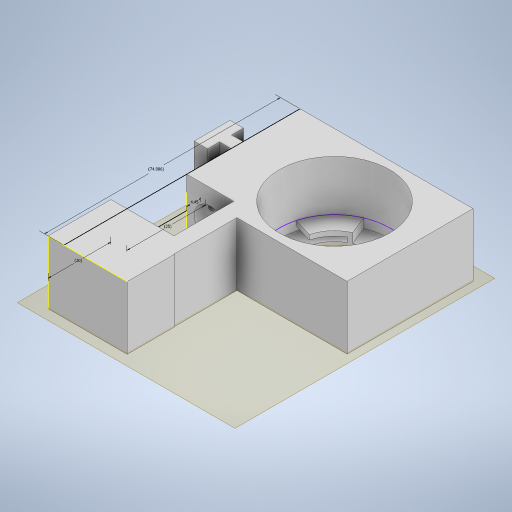
# Autodesk Inventor part: spoutextrusion
Saved by Autodesk Inventor 2023 (Build 270158000, 158)
## iProperties
Created: 2025-10-02
Part Number: spoutextrusion
Material: Generic
Document SubType Name: Modeling
Designer: ptato_qo49uko
Density: 1 g/cm^3
Appearance: Default
Author: ptato_qo49uko
Autodesk Inventor part; units mm, degrees
ref_plane "YZ Plane" through (0, 0, 0) normal (1, 0, 0) x (0, 1, 0)
ref_plane "XZ Plane" through (0, 0, 0) normal (0, 1, 0) x (-1, 0, 0)
ref_plane "XY Plane" through (0, 0, 0) normal (0, 0, 1) x (1, 0, 0)
sketch "Sketch1" plane through (0, 0, 0) normal (0, 1, 0) x (-1, 0, 0)
  line L0 (-2.2478, 1.8858) -> (1.3522, 1.8858)
  line L1 (-2.2478, 1.8858) -> (-2.2478, -1.9142)
  line L2 (-2.2478, -1.9142) -> (1.3522, -1.9142)
  line L3 (1.3522, 1.8858) -> (1.3522, 5.6858)
  line L4 (1.3522, -1.9142) -> (1.3522, -5.7142)
  line L5 (1.3522, -5.7142) -> (5.6322, -5.7142)
  line L6 (5.6322, -5.7142) -> (5.6322, 5.6858)
  line L7 (1.3522, 5.6858) -> (5.6322, 5.6858)
  point P0 (0, 0)
  dimension "d1" = 3.6
  dimension "d2" = 3.8
  dimension "d3" = 3.8
  dimension "d4" = 3.8
  dimension "d6" = 4.28
  dimension "d7" = 11.4
  dimension "d98" = 3.6
  constraints: 16 end point, 3 vertical, 2 horizontal, 2 perpendicular
  measures "d1" distance of L0.start L0.end
  measures "d2" distance of L0.start L1.end
  measures "d3" distance of L0.end L3.end
  measures "d4" distance of L2.end L4.end
  measures "d6" distance of L4.end L5.end
  measures "d7" distance of L5.end L6.end
  measures "d98" distance of L1.end L2.end
extrude "Extrusion1" add sketch "Sketch1" along normal blind 20
sketch "Sketch2" plane through (2.2478, 0, 1.8858) normal (1, 0, 0) x (0, 0, -1)
  line L0 (3.8, 0) -> (7.6, 0) projected
  line L1 (0, 20) -> (3.8, 20) projected
  line L2 (1.9, 20) -> (-18.1, 20)
  line L3 (21.9, 20) -> (1.9, 20)
  line L4 (1.8858, 0) -> (21.8858, 0)
  line L5 (0, 0) -> (3.8, 0) projected
  line L6 (1.8858, 0) -> (-18.1, 0)
  line L7 (-18.1, 0) -> (-18.1, 20)
  line L8 (21.9, 20) -> (21.8858, 0)
  point P0 (12, 0)
  point P1 (3.8, 0)
  dimension "d17" = 20
  dimension "d26" = 20
  dimension "d27" = 20
  constraints: 12 end point, 3 point on line, 2 collinear, 1 midpoint, 1 perpendicular
  measures "d17" distance of L2.start L2.end
  measures "d26" distance of L3.start L2.start
  measures "d27" distance of L4.start L4.end
extrude "Extrusion2" add sketch "Sketch2" along normal blind 55
sketch "Sketch4" plane through (0, 20, 0) normal (0, 1, 0) x (1, 0, 0)
  line L0 (2.2478, 1.9142) -> (-1.3522, 1.9142) projected
  line L1 (2.2478, -1.8858) -> (2.2478, 1.9142)
  line L2 (2.2478, 0.0142) -> (33.2478, 0.0142)
  point P0 (0, 0)
  dimension "d16" = 31
  constraints: 4 end point, 1 horizontal, 1 midpoint, 1 vertical
  measures "d16" distance of L2.start L2.end
sketch "Sketch5" plane through (0, 20, 0) normal (0, 1, 0) x (1, 0, 0)
  point P0 (0, 0)
hole "Hole2" at (33.2478, 20, -0.0142) direction (0, -1, 0) diameter 22.5 depth 22.5 counterbore diameter 35 counterbore depth 19
sketch "Sketch6" plane through (0, 0, 0) normal (0, -1, 0) x (1, 0, 0)
  point P0 (0, 0)
sketch "Sketch7" plane through (2.2478, 0, 19.9858) normal (0, 0, 1) x (1, 0, 0)
  line L0 (0, 0) -> (55, 0) projected
  line L1 (0, 0) -> (55, 0) projected
  line L2 (15, 0) -> (15, 20)
  line L3 (15, 20) -> (20, 20)
  line L4 (0, 20) -> (55, 20) projected
  line L5 (20, 20) -> (20, 0)
  line L6 (42.25, 0) -> (19.75, 0) projected
  line L7 (15, 0) -> (20, 0)
  point P0 (-2.2478, 0)
  dimension "d41" = 5
  constraints: 8 end point, 3 point on line, 1 collinear, 1 perpendicular
  measures "d41" distance of L2.end L3.end
extrude "Extrusion4" add sketch "Sketch7" along normal blind 20
sketch "Sketch10" plane through (17.2478, 0, 19.9858) normal (-1, 0, 0) x (0, 0, 1)
  line L0 (0, 20) -> (20, 20) projected
  line L1 (0, 0) -> (20, 0) projected
  line L2 (20, 20) -> (15, 20)
  line L3 (15, 20) -> (15, 0)
  line L4 (15, 0) -> (20, 0)
  line L5 (20, 0) -> (20, 20)
  point P0 (-19.9858, 0)
  point P1 (20, 0)
  dimension "d42" = 5
  constraints: 8 end point, 2 parallel, 1 horizontal, 1 perpendicular, 1 point on line
  measures "d42" distance of L4.end L3.end
extrude "Extrusion6" add sketch "Sketch10" along normal blind 20
sketch "Sketch11" plane through (2.2478, 0, 19.9858) normal (0, 0, 1) x (1, 0, 0)
  point P0 (-2.2478, 0)
sketch "Sketch12" plane through (2.2478, 0, 19.9858) normal (0, 0, 1) x (1, 0, 0)
  point P0 (-2.2478, 0)
sketch "Sketch13" plane through (2.2478, 0, 19.9858) normal (0, 0, 1) x (1, 0, 0)
  point P0 (-2.2478, 0)
sketch "Sketch14" plane through (2.2478, 0, 19.9858) normal (0, 0, 1) x (1, 0, 0)
  line L0 (0, 0) -> (15, 0) projected
  line L1 (7.5, 0) -> (7.5, 10)
  line L2 (0, 20) -> (15, 20) projected
  point P0 (-2.2478, 0)
  dimension "d45" = 10
  constraints: 2 end point, 1 midpoint, 1 perpendicular
  measures "d45" distance of L1.start L1.end
hole "Hole3" at (9.7478, 10, 19.9858) direction (0, 0, -1) diameter 10 depth 49.5
sketch "Sketch15" plane through (2.2478, 0, 39.9858) normal (0, 0, 1) x (1, 0, 0)
  line L0 (-3.6, 20) -> (-7.88, 20) projected
  line L1 (42.25, 0) -> (19.75, 0) projected
  line L2 (-5.0624, 20) -> (20.1325, 20)
  line L3 (20.1325, 20) -> (20.1325, 0)
  line L4 (20.1325, 0) -> (-5.0624, 0)
  line L5 (20, 20) -> (-5, 20) projected
  line L6 (20, 0) -> (-5, 0) projected
  line L7 (-5, 20) -> (-5, 0)
  point P0 (-2.2478, 0)
  point P1 (19.75, 0)
  constraints: 8 end point, 2 point on line, 1 horizontal, 1 parallel, 1 perpendicular
extrude "Extrusion7" add sketch "Sketch15" along normal blind 15
sketch "Sketch18" plane through (0, 20, 0) normal (0, 1, 0) x (1, 0, 0)
  line L0 (2.2478, 1.9142) -> (2.2478, 20) projected
  line L1 (2.2478, 20) -> (2.2478, -54.9858)
  line L2 (22.3802, -54.9858) -> (-2.7522, -54.9858) projected
  point P0 (0, 0)
  dimension "d73" = 74.9858
  constraints: 2 end point, 1 point on line, 1 vertical
  measures "d73" distance of L0.end L1.end
sketch "Sketch19" plane through (2.2478, 0, 1.8858) normal (-1, 0, 0) x (0, 0, 1)
  circle A0 centre (10, 10) radius 1.55 projected
  line L0 (18.1, 20) -> (18.1, 0) projected
  line L1 (18.1, 10) -> (8.1, 10)
  point P0 (-1.8858, 0)
  dimension "d75" = 10
  constraints: 2 end point, 1 horizontal, 1 midpoint
  measures "d75" distance of L1.start L1.end
hole "Hole6" at (2.2478, 10, 9.9858) direction (1, 0, 0) diameter 3.1 depth 13.5
sketch "Sketch20" plane through (2.2478, 0, 1.8858) normal (-1, 0, 0) x (0, 0, 1)
  circle A0 centre (8.1, 10) radius 1.55 projected
  line L0 (8.1, 10) -> (33.1, 10)
  line L1 (33.1, 20) -> (33.1, 0) projected
  point P0 (-1.8858, 0)
  dimension "d83" = 25
  constraints: 2 end point, 1 midpoint
  measures "d83" distance of L0.start L0.end
sketch "Sketch21" plane through (17.2478, 0, 19.9858) normal (-1, 0, 0) x (0, 0, 1)
  point P0 (-19.9858, 0)
sketch "Sketch22" plane through (0, 20, 0) normal (0, 1, 0) x (1, 0, 0)
  line L0 (2.2478, -19.9858) -> (17.2478, -19.9858) projected
  line L1 (2.2478, -19.9858) -> (17.2478, -19.9858)
  line L2 (17.2478, -19.9858) -> (17.2478, -15.9858)
  line L3 (17.2478, -15.9858) -> (2.2478, -15.9858)
  line L4 (2.2478, -15.9858) -> (2.2478, -19.9858)
  point P0 (0, 0)
  dimension "d84" = 15
  dimension "d85" = 4
  constraints: 8 end point, 2 parallel, 1 horizontal, 1 perpendicular
  measures "d84" distance of L3.end L2.end
  measures "d85" distance of L2.end L1.end
extrude "Extrusion8" cut sketch "Sketch22" against normal blind 22.25
sketch "Sketch23" plane through (17.2478, 0, 34.9858) normal (0, 0, -1) x (-1, 0, 0)
  circle A0 centre (10, 10) radius 2.5 projected
  circle A1 centre (7.5, 10) radius 3
  point P0 (17.2478, 0)
  dimension "d88" = 6
  constraints: 1 centre point, 1 horizontal alignment, 1 other
  measures "d88" diameter of A1
hole "Hole7" at (9.7478, 10, 34.9858) direction (0, 0, 1) diameter 6 depth 17
sketch "Sketch24" plane through (2.2478, 0, 1.8858) normal (-1, 0, 0) x (0, 0, 1)
  circle A0 centre (8.1, 10) radius 1.55 projected
  line L0 (9.65, 10) -> (14.1, 10)
  line L1 (14.1, 5) -> (14.1, 15) projected
  point P0 (-1.8858, 0)
  dimension "d96" = 4.45
  constraints: 2 end point, 1 horizontal alignment, 1 midpoint, 1 other
  measures "d96" distance of L0.start L0.end
sketch "Sketch25" plane through (-2.7522, 0, 19.9858) normal (-1, 0, 0) x (0, 0, 1)
  line L0 (15, 0) -> (15, 20) projected
  line L1 (15, 10) -> (35, 10)
  line L2 (35, 0) -> (35, 20) projected
  point P0 (-19.9858, 0)
  dimension "d97" = 20
  constraints: 2 end point, 2 midpoint
  measures "d97" distance of L1.start L1.end
ref_plane "Work Plane2" through (33.2478, 0.5, -0.0142) normal (0, 1, 0) x (1, 0, 0)
sketch "Sketch26" plane through (33.2478, 1, -0.0142) normal (0, 1, 0) x (1, 0, 0)
  circle A0 centre (0, 0) radius 17.5
  point P0 (-33.2478, -0.0142)
  constraints: 1 centre point
extrude "Extrusion9" add sketch "Sketch26" along normal blind 3
sketch "Sketch27" plane through (33.2478, 4, -0.0142) normal (0, 1, 0) x (1, 0, 0)
  circle A0 centre (0, 0) radius 17.5
  point P0 (-33.2478, -0.0142)
  constraints: 1 centre point
sketch "Sketch29" plane through (33.2478, 1, -0.0142) normal (0, -1, 0) x (1, 0, 0)
  circle A0 centre (0, 0) radius 17.5
  point P0 (-33.2478, 0.0142)
  constraints: 1 centre point
extrude "Extrusion10" cut sketch "Sketch29" against normal blind 1.5
sketch "Sketch30" plane through (33.2478, 2.5, -0.0142) normal (0, -1, 0) x (1, 0, 0)
  circle A0 centre (0, 0) radius 11.25
  point P0 (-33.2478, 0.0142)
  constraints: 1 centre point
extrude "Extrusion11" cut sketch "Sketch30" against normal blind 24
sketch "Sketch31" plane through (33.2478, 4, -0.0142) normal (0, 1, 0) x (1, 0, 0)
  circle A0 centre (0, 0) radius 17.5 projected
  arc A1 (16.4479, -5.9763) -> (-4.1987, 16.9888) centre (0, 0) ccw
  arc A2 (-16.8627, 4.6795) -> (5.4693, -16.6234) centre (0, 0) ccw
  line L0 (5.4693, -16.6234) -> (3.5666, -10.6697)
  circle A3 centre (0, 0) radius 11.25 projected
  line L1 (-16.8627, 4.6795) -> (-10.8414, 2.861)
  line L2 (16.4479, -5.9763) -> (10.6485, -3.6292)
  line L3 (-6.8407, 16.1076) -> (-4.502, 10.3099)
  point P0 (-33.2478, -0.0142)
  point P1 (-10.8773, 2.8718)
  point P2 (5.4693, -16.6234)
  constraints: 12 point on circle, 8 end point, 2 centre point, 1 concentric
extrude "Extrusion12" cut sketch "Sketch31" against normal blind 2.25 contours A0 L2 A3 L3 | A0 L1 A3 L0
sketch "Sketch32" plane through (33.2478, 4, -0.0142) normal (0, 1, 0) x (1, 0, 0)
  arc A0 (5.4693, -16.6234) -> (16.4479, -5.9763) centre (0, 0) ccw projected
  arc A1 (5.4693, -16.6234) -> (7.348, -15.8826) centre (0, 0) ccw
  line L0 (3.5666, -10.6697) -> (5.4693, -16.6234) projected
  line L1 (5.4693, -16.6234) -> (3.5666, -10.6697)
  line L2 (7.348, -15.8826) -> (4.9745, -10.0904)
  arc A2 (3.5666, -10.6697) -> (10.6485, -3.6292) centre (0, 0) ccw projected
  arc A3 (3.5666, -10.6697) -> (4.9745, -10.0904) centre (1.7167, -4.1725) ccw
  arc A4 (-6.8407, 16.1076) -> (-16.8627, 4.6795) centre (0, 0) ccw projected
  arc A5 (-6.8407, 16.1076) -> (-8.6833, 15.1938) centre (0, 0) ccw
  line L3 (-6.8407, 16.1076) -> (-4.502, 10.3099) projected
  line L4 (-6.8407, 16.1076) -> (-4.502, 10.3099)
  line L5 (-8.6833, 15.1938) -> (-5.6713, 9.7159)
  arc A6 (-4.502, 10.3099) -> (-10.8773, 2.8718) centre (0, 0) ccw projected
  arc A7 (-4.502, 10.3099) -> (-5.6713, 9.7159) centre (0, 0) ccw
  point P0 (-33.2478, -0.0142)
  constraints: 12 point on circle, 8 end point, 4 centre point, 2 collinear, 1 concentric
extrude "Extrusion13" add sketch "Sketch32" against normal blind 3 contours L0 A3 L2 A0 | L3 A6 L5 A4
body "Solid1"
